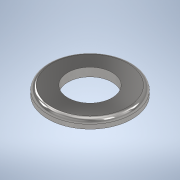
# Autodesk Inventor part: Arandela
Saved by Autodesk Inventor 2020 (Build 240168000, 168)
## iProperties
Created: 2020-09-17
Part Number: Arandela
Material: Steel AISI 1020 108 ANLD
Document SubType Name: Modeling
Designer: aaron
Density: 7.87 g/cm^3
Appearance: Steel - Polished
Author: aaron
Autodesk Inventor part; units mm, degrees
ref_plane "YZ Plane" through (0, 0, 0) normal (1, 0, 0) x (0, 1, 0)
ref_plane "XZ Plane" through (0, 0, 0) normal (0, 1, 0) x (-1, 0, 0)
ref_plane "XY Plane" through (0, 0, 0) normal (0, 0, 1) x (1, 0, 0)
sketch "Sketch1" plane through (0, 0, 0) normal (0, 1, 0) x (-1, 0, 0)
  circle A0 centre (0, 0) radius 15.875
  circle A1 centre (0, 0) radius 8.3344
  dimension "d0" = 31.75
  dimension "d1" = 16.6687
  constraints: 2 centre point, 2 coincident
  measures "d0" diameter of A0
  measures "d1" diameter of A1
extrude "Extrusion1" add sketch "Sketch1" against normal blind 3.175
fillet "Fillet2" radius 1.5875 1 edges at (15.875, 0, 0)
body "Solid1"
